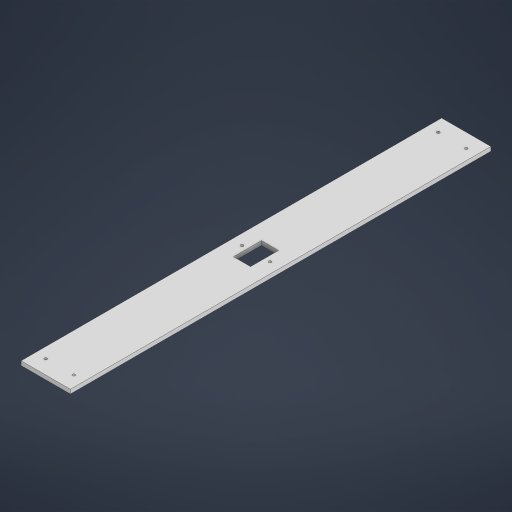
# Autodesk Inventor part: centerlegg_short_side
Saved by Autodesk Inventor 2024 (Build 280153000, 153)
## iProperties
Created: 2023-05-23
Part Number: centerlegg_short_side
Material: Generic
Document SubType Name: Modeling
Designer: aasmu
Density: 1 g/cm^3
Appearance: Default
centerlegg_plate_width: 6.000 mm
inner_carriage_length: 72.000 mm
cabel_rod_length: 25.000 mm
Author: aasmu
Autodesk Inventor part; units mm, degrees
ref_plane "YZ Plane" through (0, 0, 0) normal (1, 0, 0) x (0, 1, 0)
ref_plane "XZ Plane" through (0, 0, 0) normal (0, 1, 0) x (-1, 0, 0)
ref_plane "XY Plane" through (0, 0, 0) normal (0, 0, 1) x (1, 0, 0)
sketch "Sketch2" plane through (0, 0, 0) normal (0, 0, 1) x (1, 0, 0)
  line L0 (0, 0) -> (72, 0)
  line L1 (72, 0) -> (72, 615)
  line L2 (72, 615) -> (0, 615)
  line L3 (0, 615) -> (0, 0)
  line L4 (0, 41) -> (72, 41) construction
  line L5 (36, 41) -> (36, 0) construction
  line L6 (15.5, 20.5) -> (56.5, 20.5) construction
  circle A0 centre (15.5, 20.5) radius 2
  circle A1 centre (56.5, 20.5) radius 2
  line L7 (0, 307.5) -> (72, 307.5) construction
  circle A2 centre (15.5, 307.5) radius 2
  circle A3 centre (56.5, 307.5) radius 2
  line L8 (23.5, 328) -> (48.5, 328)
  line L9 (48.5, 328) -> (48.5, 287)
  line L10 (48.5, 287) -> (23.5, 287)
  line L11 (23.5, 287) -> (23.5, 328)
  line L12 (36, 328) -> (36, 287) construction
  circle A4 centre (15.5, 594.5) radius 2
  circle A5 centre (56.5, 594.5) radius 2
  point P0 (36, 20.5)
  point P1 (36, 307.5)
  dimension "d13" = 615
  dimension "d14" = 72
  dimension "d15" = 41
  dimension "d16" = 20.5
  dimension "d17" = 4
  dimension "d18" = 20.5
  dimension "d19" = 20.5
  dimension "d20" = 41
  dimension "d21" = 25
  constraints: 26 end point, 10 midpoint, 6 centre point, 4 parallel, 4 point on line, 3 equal radius, 3 horizontal, 3 perpendicular, 2 coincident, 2 symmetric about line, 2 other
  measures "d13" distance of L2.end L0.start
  measures "d14" distance of L0.start L0.end
  measures "d15" distance between parallel lines of L0 L4
  measures "d16" distance of point (36, 20.5) L6.start
  measures "d17" diameter of A0
  measures "d18" distance of point (36, 307.5) A2.centre
  measures "d19" distance of A3.centre point (36, 307.5)
  measures "d20" distance of L8.end L9.end
  measures "d21" distance of L9.end L10.end
extrude "Extrusion1" add sketch "Sketch2" along normal blind 6
equation "\"d13\" = centerlegg_height"
equation "\"d14\" = inner_carriage_length"
equation "\"d15\" = inner_carriage_height"
equation "\"d16\" = center_to_screw"
equation "\"d17\" = screw_size"
equation "\"d18\" = center_to_screw"
equation "\"d19\" = center_to_screw"
equation "\"d20\" = inner_carriage_height"
equation "\"d21\" = cabel_rod_length"
equation "\"d22\" = centerlegg_plate_width"
equation "\"centerlegg_plate_width\" = 6"
equation "\"centerlegg_height\" = 615"
equation "\"inner_carriage_length\" = 72"
equation "\"inner_carriage_height\" = 41"
equation "\"screw_size\" = 4"
equation "\"cabel_rod_length\" = 25"
equation "\"center_to_screw\" = 20.5"
body "Solid1"
